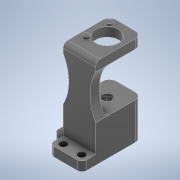
# Autodesk Inventor part: Base
Saved by Autodesk Inventor 2022 (Build 260153000, 153)
## iProperties
Created: 2021-11-22
Part Number: Base
Material: Genérico
Document SubType Name: Modeling
Designer: JK
Density: 1 g/cm^3
Appearance: Suave - Negro
Author: JK
Autodesk Inventor part; units mm, degrees
ref_plane "YZ Plane" through (0, 0, 0) normal (1, 0, 0) x (0, 1, 0)
ref_plane "XZ Plane" through (0, 0, 0) normal (0, 1, 0) x (-1, 0, 0)
ref_plane "XY Plane" through (0, 0, 0) normal (0, 0, 1) x (1, 0, 0)
sketch "Boceto1" plane through (0, 0, 0) normal (0, 1, 0) x (-1, 0, 0)
  line L0 (-7.1, 8.1) -> (7.1, 8.1)
  line L1 (7.1, 8.1) -> (7.1, -8.1)
  line L2 (7.1, -8.1) -> (-7.1, -8.1)
  line L3 (-7.1, -8.1) -> (-7.1, 8.1)
  line L4 (5.1, 6.1) -> (-5.1, 6.1)
  line L5 (-5.1, 6.1) -> (-5.1, -6.1)
  line L6 (-5.1, -6.1) -> (5.1, -6.1)
  line L7 (5.1, -6.1) -> (5.1, 6.1)
  line L8 (5.1, 6.1) -> (-5.1, -6.1) construction
  line L9 (-5.1, 6.1) -> (5.1, -6.1) construction
  point P0 (0, 0)
  point P1 (0, 0)
  point P2 (0, 0)
  point P3 (0, 0)
  point P4 (0, 0)
  point P5 (0, 0)
  dimension "d44" = 2
  dimension "d45" = 2
  dimension "d46" = 2
  dimension "d47" = 2
  dimension "d48" = 10.2
  dimension "d49" = 12.2
  constraints: 20 end point, 4 midpoint, 4 parallel, 3 coincident, 2 horizontal, 2 perpendicular
  measures "d44" distance between parallel lines of L0 L4
  measures "d45" distance between parallel lines of L2 L6
  measures "d46" distance between parallel lines of L1 L7
  measures "d47" distance between parallel lines of L3 L5
  measures "d48" distance of L4.start L4.end
  measures "d49" distance of L6.end L4.start
extrude "Extrusión1" add sketch "Boceto1" along normal blind 15
sketch "Boceto2" plane through (0, 15, 0) normal (0, 1, 0) x (1, 0, 0)
  line L0 (7.1, 8.1) -> (-7.1, 8.1) projected
  line L1 (-7.1, 8.1) -> (-7.1, -8.1) projected
  line L2 (-7.1, -8.1) -> (7.1, -8.1) projected
  line L3 (7.1, -8.1) -> (7.1, 8.1) projected
  line L4 (-5.1, -6.1) -> (-5.1, 6.1) projected
  line L5 (-5.1, 6.1) -> (5.1, 6.1) projected
  line L6 (5.1, 6.1) -> (5.1, -6.1) projected
  line L7 (5.1, -6.1) -> (-5.1, -6.1) projected
  point P0 (0, 0)
extrude "Extrusión2" add sketch "Boceto2" along normal blind 1 contours L3 L2 L1 L0 | L4 L5 L6 L7
sketch "Boceto3" plane through (0, 0, 0) normal (0, -1, 0) x (1, 0, 0)
  circle A0 centre (0, 0) radius 2.15
  line L0 (5.1, 6.1) -> (-5.1, 6.1) projected
  dimension "d10" = 4.3
  constraints: 1 centre point, 1 coincident
  measures "d10" diameter of A0
extrude "Extrusión3" cut sketch "Boceto3" against normal through all
fillet "Empalme1" radius 1.15 4 edges at (5.1, 7.5, 6.1) (5.1, 7.5, -6.1) (-5.1, 7.5, -6.1) (-5.1, 7.5, 6.1)
fillet "Empalme2" radius 3 4 edges at (7.1, 8, -8.1) (7.1, 8, 8.1) (-7.1, 8, 8.1) (-7.1, 8, -8.1)
sketch "Boceto10" plane through (0, 0, 0) normal (0, -1, 0) x (1, 0, 0)
  arc A0 (-7.1, -5.1) -> (-4.1, -8.1) centre (-4.1, -5.1) ccw projected
  line L0 (4.1, -8.1) -> (-4.1, -8.1) projected
  arc A1 (4.1, -8.1) -> (7.1, -5.1) centre (4.1, -5.1) ccw projected
  line L1 (7.1, 5.1) -> (7.1, -5.1) projected
  arc A2 (7.1, 5.1) -> (4.1, 8.1) centre (4.1, 5.1) ccw projected
  line L2 (-4.1, 8.1) -> (4.1, 8.1) projected
  arc A3 (-4.1, 8.1) -> (-7.1, 5.1) centre (-4.1, 5.1) ccw projected
  line L3 (-7.1, -5.1) -> (-7.1, 5.1) projected
  line L4 (3.95, 6.1) -> (-3.95, 6.1) projected
  arc A4 (5.1, 4.95) -> (3.95, 6.1) centre (3.95, 4.95) ccw projected
  line L5 (5.1, -4.95) -> (5.1, 4.95) projected
  arc A5 (3.95, -6.1) -> (5.1, -4.95) centre (3.95, -4.95) ccw projected
  line L6 (-3.95, -6.1) -> (3.95, -6.1) projected
  arc A6 (-5.1, -4.95) -> (-3.95, -6.1) centre (-3.95, -4.95) ccw projected
  line L7 (-5.1, 4.95) -> (-5.1, -4.95) projected
  arc A7 (-3.95, 6.1) -> (-5.1, 4.95) centre (-3.95, 4.95) ccw projected
  line L8 (-7.1, 5.1) -> (7.1, 5.1)
  line L9 (7.1, 5.1) -> (7.1, 12.1)
  line L10 (7.1, 12.1) -> (-7.1, 12.1)
  line L11 (-7.1, 12.1) -> (-7.1, 5.1)
  point P0 (0, 0)
  point P1 (7.1, 5.1)
  dimension "d50" = 4
  constraints: 8 end point, 2 parallel, 1 collinear, 1 horizontal, 1 perpendicular
  measures "d50" distance between parallel lines of L2 L10
extrude "Extrusión10" add sketch "Boceto10" against normal blind 39.1 contours L11 L10 L9 A2 L2 A3
sketch "Boceto11" plane through (0, 39.1, 0) normal (0, 1, 0) x (1, 0, 0)
  circle A0 centre (0, 0) radius 2.15 projected
  arc A1 (-4.1, 8.1) -> (-7.1, 5.1) centre (-4.1, 5.1) ccw projected
  line L0 (-7.1, 5.1) -> (-7.1, -5.1) projected
  arc A2 (-7.1, -5.1) -> (-4.1, -8.1) centre (-4.1, -5.1) ccw projected
  line L1 (-4.1, -8.1) -> (4.1, -8.1) projected
  arc A3 (4.1, -8.1) -> (7.1, -5.1) centre (4.1, -5.1) ccw projected
  line L2 (7.1, -5.1) -> (7.1, 5.1) projected
  arc A4 (7.1, 5.1) -> (4.1, 8.1) centre (4.1, 5.1) ccw projected
  line L3 (4.1, 8.1) -> (-4.1, 8.1) projected
extrude "Extrusión11" add sketch "Boceto11" against normal blind 3.9 contours A0 | L3 A4 L2 A3 L1 A2 L0 A1
sketch "Boceto12" plane through (0, 39.1, 0) normal (0, 1, 0) x (1, 0, 0)
  circle A0 centre (0, 0) radius 5.07
  dimension "d55" = 10.14
  constraints: 1 centre point, 1 coincident
  measures "d55" diameter of A0
extrude "Extrusión12" cut sketch "Boceto12" against normal blind 6
sketch "Boceto13" plane through (7.1, 0, -5.1) normal (1, 0, 0) x (0, 0, -1)
  line L0 (-10.2, 16) -> (0, 16) projected
  line L1 (-13.2, 16) -> (-13.2, 35.2) projected
  line L2 (0, 16) -> (-13.2, 16)
  line L3 (-13.2, 16) -> (-13.2, 35.2)
  line L4 (-13.2, 35.2) -> (0, 35.2)
  line L5 (0, 35.2) -> (0, 16)
  point P0 (-5.1, 0)
  point P1 (-13.2, 16)
  point P2 (-10.2, 16)
  constraints: 8 end point, 2 parallel, 1 horizontal, 1 perpendicular
extrude "Extrusión13" cut sketch "Boceto13" against normal through all
fillet "Empalme6" radius 2 3 edges at (0, 39.1, 12.1) (0, 35.2, 8.1) (0, 16, 8.1)
sketch "Boceto14" plane through (7.1, 33.2, 8.1) normal (0, 0, -1) x (-1, 0, 0)
  line L0 (11.2, 2) -> (14.2, 2) projected
  line L1 (14.2, -17.2) -> (14.2, -15.2) projected
  arc A0 (14.2, 2) -> (14.2, -17.2) centre (31.7454, -7.6) ccw
  line L2 (0, -33.2) -> (0, 3.9) projected
  arc A1 (0, -17.2) -> (0, 2) centre (-17.5454, -7.6) ccw
  line L3 (0, -15.2) -> (0, -17.2) projected
  line L4 (0, -17.2) -> (14.2, -17.2) projected
  line L5 (14.2, -17.2) -> (14.2, -15.2) projected
  line L6 (14.2, -15.2) -> (0, -15.2) projected
  line L7 (0, 0) -> (14.2, 0) projected
  line L8 (0, -15.2) -> (0, 0) projected
  line L9 (14.2, -15.2) -> (0, -15.2) projected
  line L10 (14.2, 0) -> (14.2, -15.2) projected
  line L11 (14.2, 0) -> (14.2, 2) projected
  line L12 (14.2, 2) -> (0, 2) projected
  line L13 (0, 2) -> (0, 0) projected
  line L14 (0, 0) -> (14.2, 0) projected
  point P0 (7.1, -33.2)
  point P1 (0, -31.2)
  point P2 (14.2, 2)
  dimension "d61" = 20
  constraints: 4 point on circle, 2 centre point, 2 point on line, 1 equal radius
  measures "d61" radius of A1
extrude "Extrusión14" cut sketch "Boceto14" along normal blind 10 and the other way blind 7.75 contours L11 L7 A0 | A1 L7 L2 | L7 L10 L6 A0 | L7 A1 L6 L2 | L6 L1 A0 | L6 A1 L2
sketch "Boceto16" plane through (0, 0, 0) normal (0, -1, 0) x (1, 0, 0)
  line L0 (-7.1, 12.1) -> (-7.1, -5.1) projected
  line L1 (-7.1, 10.15) -> (7.1, 10.15)
  line L2 (7.1, 10.15) -> (7.1, 18.1)
  line L3 (7.1, 18.1) -> (-7.1, 18.1)
  line L4 (-7.1, 18.1) -> (-7.1, 10.15)
  line L5 (7.1, 12.1) -> (7.1, -5.1) projected
  line L6 (4.1, -8.1) -> (-4.1, -8.1) projected
  line L7 (-7.1, 12.1) -> (-7.1, -5.1) projected
  arc A0 (-7.1, -5.1) -> (-4.1, -8.1) centre (-4.1, -5.1) ccw projected
  line L8 (4.1, -8.1) -> (-4.1, -8.1) projected
  arc A1 (4.1, -8.1) -> (7.1, -5.1) centre (4.1, -5.1) ccw projected
  line L9 (7.1, 12.1) -> (7.1, -5.1) projected
  line L10 (3.95, 6.1) -> (-3.95, 6.1) projected
  arc A2 (5.1, 4.95) -> (3.95, 6.1) centre (3.95, 4.95) ccw projected
  line L11 (5.1, -4.95) -> (5.1, 4.95) projected
  arc A3 (3.95, -6.1) -> (5.1, -4.95) centre (3.95, -4.95) ccw projected
  line L12 (-3.95, -6.1) -> (3.95, -6.1) projected
  arc A4 (-5.1, -4.95) -> (-3.95, -6.1) centre (-3.95, -4.95) ccw projected
  line L13 (-5.1, 4.95) -> (-5.1, -4.95) projected
  arc A5 (-3.95, 6.1) -> (-5.1, 4.95) centre (-3.95, 4.95) ccw projected
  line L14 (7.1, 12.1) -> (-7.1, 12.1) projected
  point P0 (0, 0)
  point P1 (7.15, 10.15)
  point P2 (7.15, -5.15)
  point P3 (4.1, -8.1)
  point P4 (-4.1, -8.1)
  point P5 (-7.15, -5.15)
  point P6 (-7.1, 10.15)
  point P7 (7.1, 10.15)
  point P8 (-7.1, 12.1)
  point P9 (7.1, 12.1)
  dimension "d122" = 6
  constraints: 8 end point, 2 parallel, 1 collinear, 1 horizontal, 1 perpendicular, 1 vertical, 1 other
  measures "d122" distance between parallel lines of L14 L3
extrude "Extrusión15" add sketch "Boceto16" against normal blind 4 contours L4 L3 L2 L14
sketch "Boceto17" plane through (0, 0, 0) normal (0, -1, 0) x (1, 0, 0)
  circle A0 centre (-4, 15.1) radius 1.65
  circle A1 centre (4, 15.1) radius 1.65
  line L0 (-7.1, 18.1) -> (-7.1, -5.1) projected
  line L1 (7.1, 18.1) -> (-7.1, 18.1) projected
  point P0 (0, 0)
  point P1 (-7.1, -5.1)
  point P2 (-7.15, 10.15)
  point P3 (-7.15, -14.15)
  point P4 (7.15, -14.15)
  point P5 (-7.1, 12.1)
  dimension "d70" = 3.3
  dimension "d119" = 4
  dimension "d120" = 4
  dimension "d123" = 3
  constraints: 2 centre point, 1 equal radius, 1 horizontal alignment, 2 other
  measures "d70" diameter of A0
  measures "d119" horizontal distance of A0.centre point (0, 0)
  measures "d120" horizontal distance of A1.centre point (0, 0)
extrude "Extrusión16" cut sketch "Boceto17" against normal through all
fillet "Empalme9" radius 2 2 edges at (-7.1, 2, 18.1) (7.1, 2, 18.1)
sketch "Boceto20" plane through (-7.1, 0, -5.1) normal (-1, 0, 0) x (0, 0, 1)
  line L0 (21.2, 0) -> (0, 0) projected
  line L1 (16.3, 0) -> (0, 0)
  line L2 (0, 0) -> (0, 2.54)
  line L3 (0, 2.54) -> (16.3, 2.54)
  line L4 (16.3, 2.54) -> (16.3, 0)
  point P0 (5.1, 0)
  point P1 (23.3, 0)
  point P2 (-3, 0)
  point P3 (0, 0)
  point P4 (15.3, 0)
  point P5 (-9, 0)
  point P6 (-7, 0)
  point P7 (17.2, 0)
  dimension "d87" = 2.54
  dimension "d88" = 16.3
  dimension "d89" = 3
  constraints: 8 end point, 2 parallel, 1 horizontal, 1 perpendicular, 2 other
  measures "d87" distance of the line from the sketch origin of L3
  measures "d88" distance between parallel lines of L4 L2
  measures "d89" distance from line of point (-3, 0) L2
extrude "Extrusión19" add sketch "Boceto20" along normal blind 5
sketch "Boceto21" plane through (0, 0, 0) normal (0, -1, 0) x (1, 0, 0)
  line L0 (-10.72, -3.4) -> (-8.08, -3.4)
  line L1 (-8.08, -3.4) -> (-8.08, 9.45)
  line L2 (-8.08, 9.45) -> (-10.72, 9.45)
  line L3 (-10.72, 9.45) -> (-10.72, -3.4)
  line L4 (-10.72, -3.4) -> (-8.08, 9.45) construction
  line L5 (-8.08, -3.4) -> (-10.72, 9.45) construction
  line L6 (-7.1, -5.1) -> (-12.1, -5.1) projected
  line L7 (-7.1, 16.1) -> (-7.1, 11.2) projected
  point P0 (0, 0)
  point P1 (-9.4, 3.025)
  point P2 (-7.15, -5.15)
  point P3 (-7.15, 18.15)
  point P4 (-7.15, -13.15)
  point P5 (-7.15, -12.15)
  point P6 (-7.1, 12.1)
  dimension "d92" = 12.85
  dimension "d93" = 1.7
  dimension "d97" = 2.64
  dimension "d98" = 2.3
  constraints: 12 end point, 2 midpoint, 2 parallel, 1 horizontal, 1 perpendicular, 2 other
  measures "d92" distance of L2.end L0.start
  measures "d97" distance of L0.start L0.end
extrude "Extrusión20" cut sketch "Boceto21" against normal blind 4
fillet "Empalme12" radius 2 3 edges at (-12.1, 1.27, -5.1) (-12.1, 1.27, 11.2) (-7.1, 1.27, 11.2)
sketch "Boceto22" plane through (0, 0, 0) normal (0, -1, 0) x (1, 0, 0)
  line L0 (-10.72, -3.4) -> (-10.72, 9.45) projected
  line L1 (-10.72, -1.01) -> (-10.22, -0.76)
  line L2 (-10.22, -0.76) -> (-10.72, -0.51)
  line L3 (-10.72, -1.01) -> (-10.72, -0.51)
  line L4 (-8.08, -3.4) -> (-10.72, -3.4) projected
  line L5 (-8.08, 9.45) -> (-8.08, -3.4) projected
  line L6 (-8.08, -1.01) -> (-8.08, -0.51)
  line L7 (-8.08, -1.01) -> (-8.58, -0.76)
  line L8 (-8.58, -0.76) -> (-8.08, -0.51)
  dimension "d101" = 0.5
  dimension "d102" = 0.5
  dimension "d103" = 2.64
  dimension "d109" = 0.5
  constraints: 12 end point, 4 point on line, 3 equal length, 1 collinear, 1 horizontal alignment
  measures "d101" distance of L2.end L1.start
  measures "d102" horizontal distance of L2.end L1.end
  measures "d103" distance from line of L4 L1.end
  measures "d109" distance of L6.end L6.start
extrude "Extrusión21" add sketch "Boceto22" against normal up to surface (2.54 mm away)
pattern_linear "Patrón rectangular1" count 4 spacing 2.54 along (0, 0, 1) of "Extrusión21"
sketch "Boceto23" plane through (0, 39.1, 0) normal (0, 1, 0) x (1, 0, 0)
  circle A0 centre (-4, 5) radius 1.2
  circle A1 centre (-4, -5) radius 1.2
  point P0 (0, 0)
  dimension "d110" = 2.4
  dimension "d111" = 4
  dimension "d112" = 5
  dimension "d113" = 5
  constraints: 2 centre point, 1 equal radius, 1 vertical alignment
  measures "d110" diameter of A0
  measures "d111" horizontal distance of point (0, 0) A0.centre
  measures "d112" vertical distance of point (0, 0) A0.centre
  measures "d113" vertical distance of point (0, 0) A1.centre
extrude "Extrusión22" add sketch "Boceto23" along normal blind 1
sketch "Boceto18" plane through (0, 0, 0) normal (0, -1, 0) x (1, 0, 0)
  arc A0 (-7.1, -5.1) -> (-4.1, -8.1) centre (-4.1, -5.1) ccw projected
  line L0 (-7.1, -5.15) -> (7.15, -5.15)
  line L1 (7.15, -5.15) -> (7.15, -12.15)
  line L2 (7.15, -12.15) -> (-7.15, -12.15)
  line L3 (-7.15, -12.15) -> (-7.15, -5.1)
  line L4 (7.15, 18.15) -> (7.15, -5.15) projected
  arc A1 (7.15, 18.15) -> (5.15, 20.15) centre (5.15, 18.15) ccw projected
  line L5 (5.15, 20.15) -> (-5.15, 20.15) projected
  arc A2 (-5.15, 20.15) -> (-7.15, 18.15) centre (-5.15, 18.15) ccw projected
  line L6 (-7.15, 18.15) -> (-7.15, -5.15) projected
  arc A3 (-7.15, -5.15) -> (-4.15, -8.15) centre (-4.15, -5.15) ccw projected
  line L7 (4.15, -8.15) -> (-4.15, -8.15) projected
  arc A4 (4.15, -8.15) -> (7.15, -5.15) centre (4.15, -5.15) ccw projected
  line L8 (7.15, 18.15) -> (7.15, -5.15) projected
  circle A5 centre (4.15, 17.15) radius 1.65 projected
  circle A6 centre (-4.15, 17.15) radius 1.65 projected
  line L9 (4, 6.15) -> (-4, 6.15) projected
  arc A7 (5.15, 5) -> (4, 6.15) centre (4, 5) ccw projected
  line L10 (5.15, -5) -> (5.15, 5) projected
  arc A8 (4, -6.15) -> (5.15, -5) centre (4, -5) ccw projected
  line L11 (-4, -6.15) -> (4, -6.15) projected
  arc A9 (-5.15, -5) -> (-4, -6.15) centre (-4, -5) ccw projected
  line L12 (-5.15, 5) -> (-5.15, -5) projected
  arc A10 (-4, 6.15) -> (-5.15, 5) centre (-4, 5) ccw projected
  point P0 (0, 0)
  point P1 (7.15, -5.15)
  point P2 (-4.15, -8.15)
  dimension "d80" = 4
  constraints: 8 end point, 2 parallel, 1 collinear, 1 horizontal, 1 perpendicular
  measures "d80" distance between parallel lines of L7 L2
sketch "Boceto19" plane through (-7.1, 16, -5.1) normal (-1, 0, 0) x (0, 0, 1)
  line L0 (-3, -11) -> (-3, 0) projected
  line L1 (-3, -11) -> (-5, -11)
  line L2 (-5, -11) -> (-5, -16)
  line L3 (-5, -16) -> (-3, -16)
  line L4 (-3, -16) -> (-3, -11)
  line L5 (23.3, -16) -> (-5, -16) projected
  point P0 (5.1, -16)
  dimension "d84" = 2
  constraints: 8 end point, 2 parallel, 1 collinear, 1 horizontal, 1 perpendicular
  measures "d84" distance between parallel lines of L4 L2
sketch "Boceto6" plane through (-7.1, 0, -5.1) normal (-1, 0, 0) x (0, 0, 1)
  line L0 (15.35, -7) -> (-5.15, -7)
  line L1 (-5.15, -7) -> (-5.15, 7)
  line L2 (-5.15, 7) -> (15.35, 7)
  line L3 (15.35, 7) -> (15.35, -7)
  line L4 (15.35, -7) -> (-5.15, 7) construction
  line L5 (-5.15, -7) -> (15.35, 7) construction
  point P0 (5.1, 0)
  dimension "d30" = 20.5
  dimension "d31" = 7
  constraints: 12 end point, 2 midpoint, 2 parallel, 1 horizontal, 1 perpendicular
  measures "d30" distance between parallel lines of L3 L1
  measures "d31" distance from line of L2 point (5.1, 0)
sketch "Boceto7" plane through (0, 16, 0) normal (0, 1, 0) x (1, 0, 0)
  circle A0 centre (0, 0) radius 2.7
  dimension "d35" = 5.4
  constraints: 1 centre point, 1 coincident
  measures "d35" diameter of A0
sketch "Boceto8" plane through (0, 0, 0) normal (0, -1, 0) x (1, 0, 0)
  line L0 (4, -13.85) -> (-4, -13.85) projected
  arc A0 (5.15, -15) -> (4, -13.85) centre (4, -15) ccw projected
  line L1 (5.15, -25) -> (5.15, -15) projected
  arc A1 (4, -26.15) -> (5.15, -25) centre (4, -25) ccw projected
  line L2 (-4, -26.15) -> (4, -26.15) projected
  arc A2 (-5.15, -25) -> (-4, -26.15) centre (-4, -25) ccw projected
  line L3 (-5.15, -15) -> (-5.15, -25) projected
  arc A3 (-4, -13.85) -> (-5.15, -15) centre (-4, -15) ccw projected
  line L4 (6.5, -10.25) -> (-6.5, -10.25) projected
  line L5 (-6.5, -25) -> (-6.5, -10.25) projected
  arc A4 (-6.5, -25) -> (-3.5, -28) centre (-3.5, -25) ccw projected
  line L6 (3.5, -28) -> (-3.5, -28) projected
  arc A5 (3.5, -28) -> (6.5, -25) centre (3.5, -25) ccw projected
  line L7 (6.5, -10.25) -> (6.5, -25) projected
  line L8 (-6.5, 10.25) -> (6.5, 10.25) projected
  line L9 (6.5, 25) -> (6.5, 10.25) projected
  arc A6 (6.5, 25) -> (3.5, 28) centre (3.5, 25) ccw projected
  line L10 (-3.5, 28) -> (3.5, 28) projected
  arc A7 (-3.5, 28) -> (-6.5, 25) centre (-3.5, 25) ccw projected
  line L11 (-6.5, 10.25) -> (-6.5, 25) projected
  line L12 (4, 26.15) -> (-4, 26.15) projected
  arc A8 (5.15, 25) -> (4, 26.15) centre (4, 25) ccw projected
  line L13 (5.15, 15) -> (5.15, 25) projected
  arc A9 (4, 13.85) -> (5.15, 15) centre (4, 15) ccw projected
  line L14 (-4, 13.85) -> (4, 13.85) projected
  arc A10 (-5.15, 15) -> (-4, 13.85) centre (-4, 15) ccw projected
  line L15 (-5.15, 25) -> (-5.15, 15) projected
  arc A11 (-4, 26.15) -> (-5.15, 25) centre (-4, 25) ccw projected
  point P0 (0, 0)
sketch "Boceto9" plane through (-6.5, 7, -10.25) normal (0, -1, 0) x (1, 0, 0)
  circle A0 centre (6.5, 10.25) radius 2.7 projected
  line L0 (13, 20.5) -> (13, 0) projected
  line L1 (0, 20.5) -> (13, 20.5) projected
  line L2 (0, 0) -> (0, 20.5) projected
  line L3 (0, 0) -> (13, 0) projected
  point P0 (6.5, 10.25)
sketch "Boceto4" plane through (0, 16, 0) normal (0, 1, 0) x (1, 0, 0)
  circle A0 centre (0, -5) radius 1.7
  circle A1 centre (0, 5) radius 1.7
  point P0 (0, 0)
  dimension "d19" = 3.4
  dimension "d25" = 5
  dimension "d26" = 5
  constraints: 2 centre point, 1 equal radius
  measures "d19" diameter of A0
  measures "d25" distance of A1.centre point (0, 0)
  measures "d26" distance of point (0, 0) A0.centre
sketch "Boceto5" plane through (0, 0, 0) normal (0, -1, 0) x (1, 0, 0)
  circle A0 centre (0, 5) radius 1.7 projected
  circle A1 centre (0, 5) radius 2.8
  circle A2 centre (0, -5) radius 1.7 projected
  circle A3 centre (0, -5) radius 2.8
  line L0 (3.2332, 5) -> (1.6166, 2.2)
  line L1 (1.6166, 2.2) -> (-1.6166, 2.2)
  line L2 (-1.6166, 2.2) -> (-3.2332, 5)
  line L3 (-3.2332, 5) -> (-1.6166, 7.8)
  line L4 (-1.6166, 7.8) -> (1.6166, 7.8)
  line L5 (1.6166, 7.8) -> (3.2332, 5)
  line L6 (3.2332, -5) -> (1.6166, -7.8)
  line L7 (1.6166, -7.8) -> (-1.6166, -7.8)
  line L8 (-1.6166, -7.8) -> (-3.2332, -5)
  line L9 (-3.2332, -5) -> (-1.6166, -2.2)
  line L10 (-1.6166, -2.2) -> (1.6166, -2.2)
  line L11 (1.6166, -2.2) -> (3.2332, -5)
  point P0 (0, 0)
  dimension "d27" = 5.6
  constraints: 24 end point, 4 coincident, 2 centre point, 2 horizontal alignment, 2 tangent, 1 equal radius, 26 other
  measures "d27" diameter of A1
